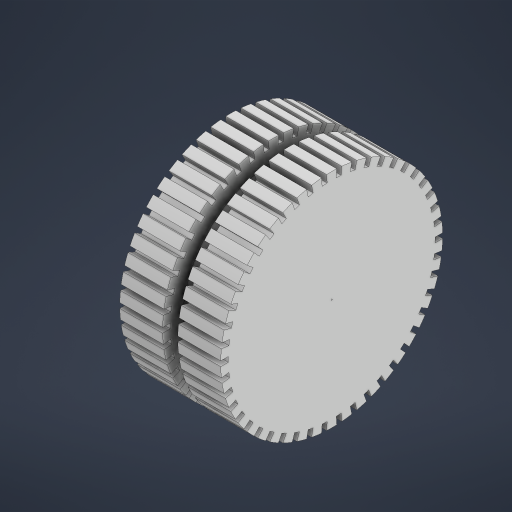
# Autodesk Inventor part: head and tail wheel
Saved by Autodesk Inventor 2024 (Build 280153000, 153)
## iProperties
Created: 2023-06-19
Part Number: head and tail wheel
Material: Generic
Document SubType Name: Modeling
Designer: dipes
Density: 1 g/cm^3
Appearance: Default
Author: dipes
Autodesk Inventor part; units mm, degrees
ref_plane "YZ Plane" through (0, 0, 0) normal (1, 0, 0) x (0, 1, 0)
ref_plane "XZ Plane" through (0, 0, 0) normal (0, 1, 0) x (-1, 0, 0)
ref_plane "XY Plane" through (0, 0, 0) normal (0, 0, 1) x (1, 0, 0)
sketch "Sketch1" plane through (0, 0, 0) normal (1, 0, 0) x (0, 1, 0)
  circle A0 centre (0, 0) radius 18
  dimension "d0" = 36
  constraints: 1 centre point, 1 coincident
  measures "d0" diameter of A0
extrude "Extrusion1" add sketch "Sketch1" along normal blind 10 and the other way blind 10
sketch "Sketch2" plane through (10, 0, 0) normal (1, 0, 0) x (0, 0, -1)
  circle A0 centre (0, 0) radius 22
  dimension "d5" = 44
  constraints: 1 centre point, 1 coincident
  measures "d5" diameter of A0
extrude "Extrusion2" add sketch "Sketch2" against normal blind 8.5
sketch "Sketch3" plane through (-10, 0, 0) normal (-1, 0, 0) x (0, 0, 1)
  circle A0 centre (0, 0) radius 22
  dimension "d8" = 44
  constraints: 1 centre point, 1 coincident
  measures "d8" diameter of A0
extrude "Extrusion3" add sketch "Sketch3" against normal blind 8.5
sketch "Sketch5" plane through (-10, 0, 0) normal (-1, 0, 0) x (0, 0, 1)
  circle A0 centre (0, 0) radius 5
  dimension "d14" = 10
  constraints: 1 centre point
  measures "d14" diameter of A0
extrude "Extrusion12" add sketch "Sketch5" along normal blind 10
sketch "Sketch14" plane through (-20, 0, 0) normal (-1, 0, 0) x (0, 0, 1)
  line L0 (-1.85, 2.75) -> (1.85, 2.75)
  line L1 (1.85, 2.75) -> (1.85, -2.75)
  line L2 (1.85, -2.75) -> (-1.85, -2.75)
  line L3 (-1.85, -2.75) -> (-1.85, 2.75)
  line L4 (-1.85, 2.75) -> (1.85, -2.75) construction
  line L5 (1.85, 2.75) -> (-1.85, -2.75) construction
  point P0 (0, 0)
  dimension "d38" = 3.7
  dimension "d39" = 5.5
  constraints: 12 end point, 2 midpoint, 2 parallel, 1 horizontal, 1 perpendicular
  measures "d38" distance of L1.end L2.end
  measures "d39" distance of L0.end L1.end
extrude "Extrusion13" cut sketch "Sketch14" against normal blind 10
sketch "Sketch15" plane through (-10, 0, 0) normal (-1, 0, 0) x (0, 0, 1)
  circle A0 centre (0, 0) radius 0.11
  dimension "d42" = 0.22
  constraints: 1 centre point, 1 coincident
  measures "d42" diameter of A0
extrude "Extrusion14" cut sketch "Sketch15" against normal blind 10
sketch "Sketch16" plane through (0, 0, 0) normal (1, 0, 0) x (0, 1, 0)
  circle A0 centre (0, 0) radius 0.11 projected
  circle A1 centre (0, 0) radius 22 construction
  line L0 (0.5, 23.5) -> (-0.5, 23.5)
  line L1 (-0.5, 23.5) -> (-0.5, 20.5)
  line L2 (-0.5, 20.5) -> (0.5, 20.5)
  line L3 (0.5, 20.5) -> (0.5, 23.5)
  circle A2 centre (0, 0) radius 22 construction
  line L4 (0.5, 23.5) -> (-0.5, 20.5) construction
  line L5 (-0.5, 23.5) -> (0.5, 20.5) construction
  line L6 (-2.7046, 23.3492) -> (-3.6953, 23.213)
  line L7 (-3.6953, 23.213) -> (-3.2868, 20.241)
  line L8 (-3.2868, 20.241) -> (-2.2961, 20.3771)
  line L9 (-2.2961, 20.3771) -> (-2.7046, 23.3492)
  line L10 (-2.7046, 23.3492) -> (-3.2868, 20.241) construction
  line L11 (-3.6953, 23.213) -> (-2.2961, 20.3771) construction
  line L12 (-5.8588, 22.7635) -> (-6.8217, 22.4937)
  line L13 (-6.8217, 22.4937) -> (-6.0123, 19.6049)
  line L14 (-6.0123, 19.6049) -> (-5.0494, 19.8747)
  line L15 (-5.0494, 19.8747) -> (-5.8588, 22.7635)
  line L16 (-5.8588, 22.7635) -> (-6.0123, 19.6049) construction
  line L17 (-6.8217, 22.4937) -> (-5.0494, 19.8747) construction
  line L18 (-8.9038, 21.7537) -> (-9.821, 21.3553)
  line L19 (-9.821, 21.3553) -> (-8.6258, 18.6036)
  line L20 (-8.6258, 18.6036) -> (-7.7086, 19.002)
  line L21 (-7.7086, 19.002) -> (-8.9038, 21.7537)
  line L22 (-8.9038, 21.7537) -> (-8.6258, 18.6036) construction
  line L23 (-9.821, 21.3553) -> (-7.7086, 19.002) construction
  line L24 (-11.783, 20.3386) -> (-12.6374, 19.8191)
  line L25 (-12.6374, 19.8191) -> (-11.0787, 17.2558)
  line L26 (-11.0787, 17.2558) -> (-10.2243, 17.7754)
  line L27 (-10.2243, 17.7754) -> (-11.783, 20.3386)
  line L28 (-11.783, 20.3386) -> (-11.0787, 17.2558) construction
  line L29 (-12.6374, 19.8191) -> (-10.2243, 17.7754) construction
  line L30 (-14.4427, 18.5448) -> (-15.2184, 17.9137)
  line L31 (-15.2184, 17.9137) -> (-13.3252, 15.5865)
  line L32 (-13.3252, 15.5865) -> (-12.5494, 16.2176)
  line L33 (-12.5494, 16.2176) -> (-14.4427, 18.5448)
  line L34 (-14.4427, 18.5448) -> (-13.3252, 15.5865) construction
  line L35 (-15.2184, 17.9137) -> (-12.5494, 16.2176) construction
  line L36 (-16.8334, 16.4054) -> (-17.5159, 15.6746)
  line L37 (-17.5159, 15.6746) -> (-15.3234, 13.6269)
  line L38 (-15.3234, 13.6269) -> (-14.6409, 14.3578)
  line L39 (-14.6409, 14.3578) -> (-16.8334, 16.4054)
  line L40 (-16.8334, 16.4054) -> (-15.3234, 13.6269) construction
  line L41 (-17.5159, 15.6746) -> (-14.6409, 14.3578) construction
  line L42 (-18.9105, 13.9605) -> (-19.4871, 13.1435)
  line L43 (-19.4871, 13.1435) -> (-17.0362, 11.4135)
  line L44 (-17.0362, 11.4135) -> (-16.4595, 12.2304)
  line L45 (-16.4595, 12.2304) -> (-18.9105, 13.9605)
  line L46 (-18.9105, 13.9605) -> (-17.0362, 11.4135) construction
  line L47 (-19.4871, 13.1435) -> (-16.4595, 12.2304) construction
  line L48 (-20.6353, 11.2555) -> (-21.0953, 10.3676)
  line L49 (-21.0953, 10.3676) -> (-18.4317, 8.9874)
  line L50 (-18.4317, 8.9874) -> (-17.9716, 9.8753)
  line L51 (-17.9716, 9.8753) -> (-20.6353, 11.2555)
  line L52 (-20.6353, 11.2555) -> (-18.4317, 8.9874) construction
  line L53 (-21.0953, 10.3676) -> (-17.9716, 9.8753) construction
  line L54 (-21.9757, 8.3408) -> (-22.3106, 7.3985)
  line L55 (-22.3106, 7.3985) -> (-19.4838, 6.3939)
  line L56 (-19.4838, 6.3939) -> (-19.1489, 7.3362)
  line L57 (-19.1489, 7.3362) -> (-21.9757, 8.3408)
  line L58 (-21.9757, 8.3408) -> (-19.4838, 6.3939) construction
  line L59 (-22.3106, 7.3985) -> (-19.1489, 7.3362) construction
  line L60 (-22.9067, 5.2708) -> (-23.1102, 4.2917)
  line L61 (-23.1102, 4.2917) -> (-20.173, 3.6813)
  line L62 (-20.173, 3.6813) -> (-19.9695, 4.6604)
  line L63 (-19.9695, 4.6604) -> (-22.9067, 5.2708)
  line L64 (-22.9067, 5.2708) -> (-20.173, 3.6813) construction
  line L65 (-23.1102, 4.2917) -> (-19.9695, 4.6604) construction
  line L66 (-23.4111, 2.1025) -> (-23.4793, 1.1049)
  line L67 (-23.4793, 1.1049) -> (-20.4863, 0.9001)
  line L68 (-20.4863, 0.9001) -> (-20.4181, 1.8978)
  line L69 (-20.4181, 1.8978) -> (-23.4111, 2.1025)
  line L70 (-23.4111, 2.1025) -> (-20.4863, 0.9001) construction
  line L71 (-23.4793, 1.1049) -> (-20.4181, 1.8978) construction
  line L72 (-23.4793, -1.1049) -> (-23.4111, -2.1025)
  line L73 (-23.4111, -2.1025) -> (-20.4181, -1.8978)
  line L74 (-20.4181, -1.8978) -> (-20.4863, -0.9001)
  line L75 (-20.4863, -0.9001) -> (-23.4793, -1.1049)
  line L76 (-23.4793, -1.1049) -> (-20.4181, -1.8978) construction
  line L77 (-23.4111, -2.1025) -> (-20.4863, -0.9001) construction
  line L78 (-23.1102, -4.2917) -> (-22.9067, -5.2708)
  line L79 (-22.9067, -5.2708) -> (-19.9695, -4.6604)
  line L80 (-19.9695, -4.6604) -> (-20.173, -3.6813)
  line L81 (-20.173, -3.6813) -> (-23.1102, -4.2917)
  line L82 (-23.1102, -4.2917) -> (-19.9695, -4.6604) construction
  line L83 (-22.9067, -5.2708) -> (-20.173, -3.6813) construction
  line L84 (-22.3106, -7.3985) -> (-21.9757, -8.3408)
  line L85 (-21.9757, -8.3408) -> (-19.1489, -7.3362)
  line L86 (-19.1489, -7.3362) -> (-19.4838, -6.3939)
  line L87 (-19.4838, -6.3939) -> (-22.3106, -7.3985)
  line L88 (-22.3106, -7.3985) -> (-19.1489, -7.3362) construction
  line L89 (-21.9757, -8.3408) -> (-19.4838, -6.3939) construction
  line L90 (-21.0953, -10.3676) -> (-20.6353, -11.2555)
  line L91 (-20.6353, -11.2555) -> (-17.9716, -9.8753)
  line L92 (-17.9716, -9.8753) -> (-18.4317, -8.9874)
  line L93 (-18.4317, -8.9874) -> (-21.0953, -10.3676)
  line L94 (-21.0953, -10.3676) -> (-17.9716, -9.8753) construction
  line L95 (-20.6353, -11.2555) -> (-18.4317, -8.9874) construction
  line L96 (-19.4871, -13.1435) -> (-18.9105, -13.9605)
  line L97 (-18.9105, -13.9605) -> (-16.4595, -12.2304)
  line L98 (-16.4595, -12.2304) -> (-17.0362, -11.4135)
  line L99 (-17.0362, -11.4135) -> (-19.4871, -13.1435)
  line L100 (-19.4871, -13.1435) -> (-16.4595, -12.2304) construction
  line L101 (-18.9105, -13.9605) -> (-17.0362, -11.4135) construction
  line L102 (-17.5159, -15.6746) -> (-16.8334, -16.4054)
  line L103 (-16.8334, -16.4054) -> (-14.6409, -14.3578)
  line L104 (-14.6409, -14.3578) -> (-15.3234, -13.6269)
  line L105 (-15.3234, -13.6269) -> (-17.5159, -15.6746)
  line L106 (-17.5159, -15.6746) -> (-14.6409, -14.3578) construction
  line L107 (-16.8334, -16.4054) -> (-15.3234, -13.6269) construction
  line L108 (-15.2184, -17.9137) -> (-14.4427, -18.5448)
  line L109 (-14.4427, -18.5448) -> (-12.5494, -16.2176)
  line L110 (-12.5494, -16.2176) -> (-13.3252, -15.5865)
  line L111 (-13.3252, -15.5865) -> (-15.2184, -17.9137)
  line L112 (-15.2184, -17.9137) -> (-12.5494, -16.2176) construction
  line L113 (-14.4427, -18.5448) -> (-13.3252, -15.5865) construction
  line L114 (-12.6374, -19.8191) -> (-11.783, -20.3386)
  line L115 (-11.783, -20.3386) -> (-10.2243, -17.7754)
  line L116 (-10.2243, -17.7754) -> (-11.0787, -17.2558)
  line L117 (-11.0787, -17.2558) -> (-12.6374, -19.8191)
  line L118 (-12.6374, -19.8191) -> (-10.2243, -17.7754) construction
  line L119 (-11.783, -20.3386) -> (-11.0787, -17.2558) construction
  line L120 (-9.821, -21.3553) -> (-8.9038, -21.7537)
  line L121 (-8.9038, -21.7537) -> (-7.7086, -19.002)
  line L122 (-7.7086, -19.002) -> (-8.6258, -18.6036)
  line L123 (-8.6258, -18.6036) -> (-9.821, -21.3553)
  line L124 (-9.821, -21.3553) -> (-7.7086, -19.002) construction
  line L125 (-8.9038, -21.7537) -> (-8.6258, -18.6036) construction
  line L126 (-6.8217, -22.4937) -> (-5.8588, -22.7635)
  line L127 (-5.8588, -22.7635) -> (-5.0494, -19.8747)
  line L128 (-5.0494, -19.8747) -> (-6.0123, -19.6049)
  line L129 (-6.0123, -19.6049) -> (-6.8217, -22.4937)
  line L130 (-6.8217, -22.4937) -> (-5.0494, -19.8747) construction
  line L131 (-5.8588, -22.7635) -> (-6.0123, -19.6049) construction
  line L132 (-3.6953, -23.213) -> (-2.7046, -23.3492)
  line L133 (-2.7046, -23.3492) -> (-2.2961, -20.3771)
  line L134 (-2.2961, -20.3771) -> (-3.2868, -20.241)
  line L135 (-3.2868, -20.241) -> (-3.6953, -23.213)
  line L136 (-3.6953, -23.213) -> (-2.2961, -20.3771) construction
  line L137 (-2.7046, -23.3492) -> (-3.2868, -20.241) construction
  line L138 (-0.5, -23.5) -> (0.5, -23.5)
  line L139 (0.5, -23.5) -> (0.5, -20.5)
  line L140 (0.5, -20.5) -> (-0.5, -20.5)
  line L141 (-0.5, -20.5) -> (-0.5, -23.5)
  line L142 (-0.5, -23.5) -> (0.5, -20.5) construction
  line L143 (0.5, -23.5) -> (-0.5, -20.5) construction
  line L144 (2.7046, -23.3492) -> (3.6953, -23.213)
  line L145 (3.6953, -23.213) -> (3.2868, -20.241)
  line L146 (3.2868, -20.241) -> (2.2961, -20.3771)
  line L147 (2.2961, -20.3771) -> (2.7046, -23.3492)
  line L148 (2.7046, -23.3492) -> (3.2868, -20.241) construction
  line L149 (3.6953, -23.213) -> (2.2961, -20.3771) construction
  line L150 (5.8588, -22.7635) -> (6.8217, -22.4937)
  line L151 (6.8217, -22.4937) -> (6.0123, -19.6049)
  line L152 (6.0123, -19.6049) -> (5.0494, -19.8747)
  line L153 (5.0494, -19.8747) -> (5.8588, -22.7635)
  line L154 (5.8588, -22.7635) -> (6.0123, -19.6049) construction
  line L155 (6.8217, -22.4937) -> (5.0494, -19.8747) construction
  line L156 (8.9038, -21.7537) -> (9.821, -21.3553)
  line L157 (9.821, -21.3553) -> (8.6258, -18.6036)
  line L158 (8.6258, -18.6036) -> (7.7086, -19.002)
  line L159 (7.7086, -19.002) -> (8.9038, -21.7537)
  line L160 (8.9038, -21.7537) -> (8.6258, -18.6036) construction
  line L161 (9.821, -21.3553) -> (7.7086, -19.002) construction
  line L162 (11.783, -20.3386) -> (12.6374, -19.8191)
  line L163 (12.6374, -19.8191) -> (11.0787, -17.2558)
  line L164 (11.0787, -17.2558) -> (10.2243, -17.7754)
  line L165 (10.2243, -17.7754) -> (11.783, -20.3386)
  line L166 (11.783, -20.3386) -> (11.0787, -17.2558) construction
  line L167 (12.6374, -19.8191) -> (10.2243, -17.7754) construction
  line L168 (14.4427, -18.5448) -> (15.2184, -17.9137)
  line L169 (15.2184, -17.9137) -> (13.3252, -15.5865)
  line L170 (13.3252, -15.5865) -> (12.5494, -16.2176)
  line L171 (12.5494, -16.2176) -> (14.4427, -18.5448)
  line L172 (14.4427, -18.5448) -> (13.3252, -15.5865) construction
  line L173 (15.2184, -17.9137) -> (12.5494, -16.2176) construction
  line L174 (16.8334, -16.4054) -> (17.5159, -15.6746)
  line L175 (17.5159, -15.6746) -> (15.3234, -13.6269)
  line L176 (15.3234, -13.6269) -> (14.6409, -14.3578)
  line L177 (14.6409, -14.3578) -> (16.8334, -16.4054)
  line L178 (16.8334, -16.4054) -> (15.3234, -13.6269) construction
  line L179 (17.5159, -15.6746) -> (14.6409, -14.3578) construction
  line L180 (18.9105, -13.9605) -> (19.4871, -13.1435)
  line L181 (19.4871, -13.1435) -> (17.0362, -11.4135)
  line L182 (17.0362, -11.4135) -> (16.4595, -12.2304)
  line L183 (16.4595, -12.2304) -> (18.9105, -13.9605)
  line L184 (18.9105, -13.9605) -> (17.0362, -11.4135) construction
  line L185 (19.4871, -13.1435) -> (16.4595, -12.2304) construction
  line L186 (20.6353, -11.2555) -> (21.0953, -10.3676)
  line L187 (21.0953, -10.3676) -> (18.4317, -8.9874)
  line L188 (18.4317, -8.9874) -> (17.9716, -9.8753)
  line L189 (17.9716, -9.8753) -> (20.6353, -11.2555)
  line L190 (20.6353, -11.2555) -> (18.4317, -8.9874) construction
  line L191 (21.0953, -10.3676) -> (17.9716, -9.8753) construction
  line L192 (21.9757, -8.3408) -> (22.3106, -7.3985)
  line L193 (22.3106, -7.3985) -> (19.4838, -6.3939)
  line L194 (19.4838, -6.3939) -> (19.1489, -7.3362)
  line L195 (19.1489, -7.3362) -> (21.9757, -8.3408)
  line L196 (21.9757, -8.3408) -> (19.4838, -6.3939) construction
  line L197 (22.3106, -7.3985) -> (19.1489, -7.3362) construction
  line L198 (22.9067, -5.2708) -> (23.1102, -4.2917)
  line L199 (23.1102, -4.2917) -> (20.173, -3.6813)
  line L200 (20.173, -3.6813) -> (19.9695, -4.6604)
  line L201 (19.9695, -4.6604) -> (22.9067, -5.2708)
  line L202 (22.9067, -5.2708) -> (20.173, -3.6813) construction
  line L203 (23.1102, -4.2917) -> (19.9695, -4.6604) construction
  line L204 (23.4111, -2.1025) -> (23.4793, -1.1049)
  line L205 (23.4793, -1.1049) -> (20.4863, -0.9001)
  line L206 (20.4863, -0.9001) -> (20.4181, -1.8978)
  line L207 (20.4181, -1.8978) -> (23.4111, -2.1025)
  line L208 (23.4111, -2.1025) -> (20.4863, -0.9001) construction
  line L209 (23.4793, -1.1049) -> (20.4181, -1.8978) construction
  line L210 (23.4793, 1.1049) -> (23.4111, 2.1025)
  line L211 (23.4111, 2.1025) -> (20.4181, 1.8978)
  line L212 (20.4181, 1.8978) -> (20.4863, 0.9001)
  line L213 (20.4863, 0.9001) -> (23.4793, 1.1049)
  line L214 (23.4793, 1.1049) -> (20.4181, 1.8978) construction
  line L215 (23.4111, 2.1025) -> (20.4863, 0.9001) construction
  line L216 (23.1102, 4.2917) -> (22.9067, 5.2708)
  line L217 (22.9067, 5.2708) -> (19.9695, 4.6604)
  line L218 (19.9695, 4.6604) -> (20.173, 3.6813)
  line L219 (20.173, 3.6813) -> (23.1102, 4.2917)
  line L220 (23.1102, 4.2917) -> (19.9695, 4.6604) construction
  line L221 (22.9067, 5.2708) -> (20.173, 3.6813) construction
  line L222 (22.3106, 7.3985) -> (21.9757, 8.3408)
  line L223 (21.9757, 8.3408) -> (19.1489, 7.3362)
  line L224 (19.1489, 7.3362) -> (19.4838, 6.3939)
  line L225 (19.4838, 6.3939) -> (22.3106, 7.3985)
  line L226 (22.3106, 7.3985) -> (19.1489, 7.3362) construction
  line L227 (21.9757, 8.3408) -> (19.4838, 6.3939) construction
  line L228 (21.0953, 10.3676) -> (20.6353, 11.2555)
  line L229 (20.6353, 11.2555) -> (17.9716, 9.8753)
  line L230 (17.9716, 9.8753) -> (18.4317, 8.9874)
  line L231 (18.4317, 8.9874) -> (21.0953, 10.3676)
  line L232 (21.0953, 10.3676) -> (17.9716, 9.8753) construction
  line L233 (20.6353, 11.2555) -> (18.4317, 8.9874) construction
  line L234 (19.4871, 13.1435) -> (18.9105, 13.9605)
  line L235 (18.9105, 13.9605) -> (16.4595, 12.2304)
  line L236 (16.4595, 12.2304) -> (17.0362, 11.4135)
  line L237 (17.0362, 11.4135) -> (19.4871, 13.1435)
  line L238 (19.4871, 13.1435) -> (16.4595, 12.2304) construction
  line L239 (18.9105, 13.9605) -> (17.0362, 11.4135) construction
  line L240 (17.5159, 15.6746) -> (16.8334, 16.4054)
  line L241 (16.8334, 16.4054) -> (14.6409, 14.3578)
  line L242 (14.6409, 14.3578) -> (15.3234, 13.6269)
  line L243 (15.3234, 13.6269) -> (17.5159, 15.6746)
  line L244 (17.5159, 15.6746) -> (14.6409, 14.3578) construction
  line L245 (16.8334, 16.4054) -> (15.3234, 13.6269) construction
  line L246 (15.2184, 17.9137) -> (14.4427, 18.5448)
  line L247 (14.4427, 18.5448) -> (12.5494, 16.2176)
  line L248 (12.5494, 16.2176) -> (13.3252, 15.5865)
  line L249 (13.3252, 15.5865) -> (15.2184, 17.9137)
  line L250 (15.2184, 17.9137) -> (12.5494, 16.2176) construction
  line L251 (14.4427, 18.5448) -> (13.3252, 15.5865) construction
  line L252 (12.6374, 19.8191) -> (11.783, 20.3386)
  line L253 (11.783, 20.3386) -> (10.2243, 17.7754)
  line L254 (10.2243, 17.7754) -> (11.0787, 17.2558)
  line L255 (11.0787, 17.2558) -> (12.6374, 19.8191)
  line L256 (12.6374, 19.8191) -> (10.2243, 17.7754) construction
  line L257 (11.783, 20.3386) -> (11.0787, 17.2558) construction
  line L258 (9.821, 21.3553) -> (8.9038, 21.7537)
  line L259 (8.9038, 21.7537) -> (7.7086, 19.002)
  line L260 (7.7086, 19.002) -> (8.6258, 18.6036)
  line L261 (8.6258, 18.6036) -> (9.821, 21.3553)
  line L262 (9.821, 21.3553) -> (7.7086, 19.002) construction
  line L263 (8.9038, 21.7537) -> (8.6258, 18.6036) construction
  line L264 (6.8217, 22.4937) -> (5.8588, 22.7635)
  line L265 (5.8588, 22.7635) -> (5.0494, 19.8747)
  line L266 (5.0494, 19.8747) -> (6.0123, 19.6049)
  line L267 (6.0123, 19.6049) -> (6.8217, 22.4937)
  line L268 (6.8217, 22.4937) -> (5.0494, 19.8747) construction
  line L269 (5.8588, 22.7635) -> (6.0123, 19.6049) construction
  line L270 (3.6953, 23.213) -> (2.7046, 23.3492)
  line L271 (2.7046, 23.3492) -> (2.2961, 20.3771)
  line L272 (2.2961, 20.3771) -> (3.2868, 20.241)
  line L273 (3.2868, 20.241) -> (3.6953, 23.213)
  line L274 (3.6953, 23.213) -> (2.2961, 20.3771) construction
  line L275 (2.7046, 23.3492) -> (3.2868, 20.241) construction
  point P0 (0, 22)
  point P1 (-2.9957, 21.7951)
  point P2 (-5.9355, 21.1842)
  point P3 (-8.7648, 20.1786)
  point P4 (-11.4308, 18.7972)
  point P5 (-13.8839, 17.0656)
  point P6 (-16.0784, 15.0162)
  point P7 (-17.9733, 12.687)
  point P8 (-19.5335, 10.1214)
  point P9 (-20.7297, 7.3674)
  point P10 (-21.5398, 4.476)
  point P11 (-21.9487, 1.5013)
  point P12 (-21.9487, -1.5013)
  point P13 (-21.5398, -4.476)
  point P14 (-20.7297, -7.3674)
  point P15 (-19.5335, -10.1214)
  point P16 (-17.9733, -12.687)
  point P17 (-16.0784, -15.0162)
  point P18 (-13.8839, -17.0656)
  point P19 (-11.4308, -18.7972)
  point P20 (-8.7648, -20.1786)
  point P21 (-5.9355, -21.1842)
  point P22 (-2.9957, -21.7951)
  point P23 (0, -22)
  point P24 (2.9957, -21.7951)
  point P25 (5.9355, -21.1842)
  point P26 (8.7648, -20.1786)
  point P27 (11.4308, -18.7972)
  point P28 (13.8839, -17.0656)
  point P29 (16.0784, -15.0162)
  point P30 (17.9733, -12.687)
  point P31 (19.5335, -10.1214)
  point P32 (20.7297, -7.3674)
  point P33 (21.5398, -4.476)
  point P34 (21.9487, -1.5013)
  point P35 (21.9487, 1.5013)
  point P36 (21.5398, 4.476)
  point P37 (20.7297, 7.3674)
  point P38 (19.5335, 10.1214)
  point P39 (17.9733, 12.687)
  point P40 (16.0784, 15.0162)
  point P41 (13.8839, 17.0656)
  point P42 (11.4308, 18.7972)
  point P43 (8.7648, 20.1786)
  point P44 (5.9355, 21.1842)
  point P45 (2.9957, 21.7951)
  dimension "d45" = 44
  dimension "d46" = 1
  dimension "d47" = 3
  dimension "d52" = 360
  constraints: 552 end point, 3 coincident, 2 midpoint, 2 parallel, 1 centre point, 1 horizontal, 1 perpendicular, 1 vertical alignment, 598 other
  measures "d45" diameter of A1
  measures "d46" distance of L2.end L1.end
  measures "d47" distance of L1.end L0.end
extrude "Extrusion15" cut sketch "Sketch16" along normal through all both and the other way through all
body "Solid1"
